Autodesk Inventor part; units mm, degrees
note: some values were not read from the file. Chosen so that the rebuilt part matches the saved one: sketch regions of "Extrusion1".
(part 2 of 2)
extrude "Extrusion3" cut sketch "Sketch3" against normal blind 0.5 contours S0 S1 S2 S3 S4 S5 S6 S7 | L16 L17 S14 S15 S16 S17 S18 S19 L18 L19 S20 S21 S22 S23 S24 L20 L21 | S25 S26 S27 S28 S29 S30 S31 S32 | S39 S40 L22 L23 L24 L25 L26 S41 S42 | S47 S48 S49 S50 L28 L29 S51 S52 S53 L30 L31 S54 S55 | L33 L34 S60 S61 S62 L35 L36 L37 L38 L39 S63 S64 L40 | S65 S66 S67 S68 S69 S70 S71 S72 | L41 L42 L43 L44 L45 L46 L47 L48 L49 L50 L51 L52 | L53 L54 L55 L56 L57 L58 L59 L60 | L61 L62 L63 L64 L65 L66 L67 | L68 L69 L70 L71 | S79 S80 S81 S82 S83 S84 L72 L73 S85 S86 S87 S88 S89 S90 S91 S92 L74 L75 S93 S94 | L76 L77 L78 L79 L80 L81 L82 L83 | L87 L88 L89 L90 L91 L92 | L93 L94 L95 L96 L97 L98 L99 L100 L101 L102 L103 L104 | S95 S96 L105 L106 L107 S97 S98 S99 L108 S100 | L115 L126 L122 | L122 L126 L127 L128 L129 L130 L131 L132 L133 | L115 L116 L117 L118 L119 L120 L121 S109 S110 S111 L122 L126 | L137 L138 L139 L140 L141 L142 L143 L144 | L145 L146 L147 L148 L149 L150 L151 L152 L153 L154 L155 L156 | S116 S117 S118 S119 S120 S121 S122 S123 | L157 L158 L159 L160 L161 L162 L163 L164 L165 L166 | L167 L168 L169 L170 L171 L172 S130 L173 L174 L175 L176 | S131 S132 S133 S134 | S143 S144 S145 S146 | S155 S156 S157 S158 | S159 S160 S161 S162 | L177 L178 L179 L180 | L181 L182 L183 L184 L185 L186 L187 | L188 L189 L190 L191 | L192 L193 L194 L195 | L196 L197 L198 L199 L200 L201 L202 | L203 L204 L205 L206 L207 L208 L209 L210 L211 L212 L213 L214 L215 | L216 L217 L218 L219 L220 L221 L222 L223 L224 L225 L226 L227 | L228 L229 L230 L231 L232 L233 L234 L235 | S171 L239 L240 S172 S173 S174 S175 S176 S177 S178 S179 L241 L242 S180 S181 S182 S183 S184 S185 S186 | S187 S188 L243 L244 L245 S189 S190 S191 S192 L246 L247 L248 S193 S194 | L249 L250 L251 L252 L253 L254 L255 S195 S196 S197 L256 | L260 L261 L262 L263 L264 L265 L266 L267 L268 L269 L270 L271 | L272 L273 L274 L275 L276 L277 L278 L279 L280 L281 L282 L283 L284 | L285 L286 L287 L288 L289 L290 L291 L292 L293 L294 L295 L296 | L297 L298 L299 L300 L301 L302 L303 L304 L305 L306 | L307 L308 L309 L310 L311 L312 L313 L314 | L315 L316 L317 L318 | L319 L320 L321 L322 L323 L324 L325
body "Solid1"
